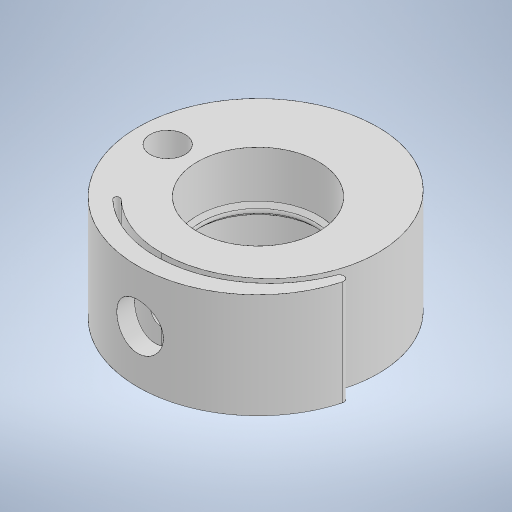
# Autodesk Inventor part: Spool
Saved by Autodesk Inventor 2023.4 (Build 274418000, 418)
## iProperties
Created: 2024-05-13
Part Number: Spool
Material: Generic
Document SubType Name: Modeling
Designer: Nathan Cai
Density: 1 g/cm^3
Appearance: Default
Author: Nathan Cai
Autodesk Inventor part; units mm, degrees
ref_plane "YZ Plane" through (0, 0, 0) normal (1, 0, 0) x (0, 1, 0)
ref_plane "XZ Plane" through (0, 0, 0) normal (0, 1, 0) x (-1, 0, 0)
sketch "Sketch1" plane through (0, 0, 0) normal (1, 0, 0) x (0, 1, 0)
  line L0 (0, 0) -> (9, 0)
  line L1 (9, 0) -> (9, -10.3188)
  line L2 (9, -10.3188) -> (0, -10.3188)
  line L3 (0, -10.3188) -> (0, 0)
  line L4 (9, 0) -> (0, 0)
  line L5 (0, 0) -> (0, -5.2)
  line L6 (0, -5.2) -> (9, -5.2)
  line L7 (9, -5.2) -> (9, 0)
  line L8 (5, -5.2) -> (4, -5.2)
  line L9 (4, -5.2) -> (4, -4.7)
  line L10 (4, -4.7) -> (5, -4.7)
  line L11 (5, -4.7) -> (5, -5.2)
  dimension "d0" = 9
  dimension "d1" = 5.2
  dimension "d2" = 10.3187
  dimension "d3" = 0.5
  dimension "d4" = 4
  dimension "d5" = 4
  constraints: 24 end point, 6 parallel, 3 horizontal, 3 perpendicular, 2 point on line
  measures "d0" distance of L1.end L2.end
  measures "d1" distance of L5.end L4.end
  measures "d2" distance between parallel lines of L0 L2
  measures "d3" distance of L8.end L9.end
  measures "d4" distance between parallel lines of L3 L9
  measures "d5" distance between parallel lines of L1 L11
revolve "Revolution1" add sketch "Sketch1" angle 360 about axis through (0, 0, 0) along (0, 1, 0) contours L6 L1 L2 L3 | L9 L10 L11 L6
chamfer "Chamfer1" distance 0.5 angle 45 2 edges at (0, 4, 4.7) (0, 5, 4.7)
fillet "Fillet1" radius 0.25 2 edges at (0, 4.4999, 4.7) (0, 4.5001, 4.7)
sketch "Sketch2" plane through (0, 9, 0) normal (0, 1, 0) x (1, 0, 0)
  circle A0 centre (0, 0) radius 5.2 projected
  line L0 (-5.2, 0) -> (-10.3188, 0) construction
  circle A1 centre (-7.7594, 0) radius 1.5
  circle A2 centre (0, 0) radius 10.3188 projected
  line L1 (0, 0) -> (0, -10.3188) construction
  arc A3 (0, -8.3188) -> (0, 10.3188) centre (0, 1) ccw
  arc A4 (-5.8822, -5.8822) -> (0, -8.3188) centre (0, 0) ccw
  line L2 (-5.8822, -5.8822) -> (-7.2965, -7.2965)
  arc A5 (0, -8.8268) -> (0, 10.8268) centre (0, 1) ccw
  arc A6 (-6.2415, -6.2415) -> (0, -8.8268) centre (0, 0) ccw
  point P0 (8.7585, 5.4558)
  dimension "d11" = 3
  dimension "d14" = 2
  dimension "d15" = 45
  dimension "d22" = 0.508
  constraints: 12 point on circle, 6 end point, 5 centre point, 4 point on line, 2 tangent, 1 concentric, 1 horizontal, 1 horizontal alignment, 1 line through centre, 1 midpoint, 1 vertical, 1 other
  measures "d11" diameter of A1
  measures "d14" distance of L1.end A3.start
  measures "d15" angle of L1 L2
  measures "d22" radial gap between concentric circles of A3 A5
extrude "Extrusion1" cut sketch "Sketch2" against normal through all contours A1 | A2 A5 A6 L2 A4 A3
sketch "Sketch3" plane through (0, 0, 0) normal (0, 0, 1) x (1, 0, 0)
  line L0 (5.2, 9) -> (-5.2, 9) projected
  line L1 (0, 9) -> (0, 0) construction
  circle A0 centre (0, 4.5) radius 1
  dimension "d16" = 2
  constraints: 2 end point, 2 midpoint, 1 centre point, 1 vertical
  measures "d16" diameter of A0
extrude "Extrusion2" cut sketch "Sketch3" along normal through all
fillet "Fillet2" radius 0.4 1 edges at (8.7585, 4.5, -5.4558)
fillet "Fillet3" radius 0.254 2 edges at (-6.2415, 4.5, 6.2415) (-5.8822, 4.5, 5.8822)
ref_plane "Work Plane1" through (0, 0, 11.1125) normal (0, 0, 1) x (1, 0, 0)
sketch "Sketch4" plane through (0, 0, 11.1125) normal (0, 0, 1) x (1, 0, 0)
  line L0 (0, 9) -> (0, 0) construction
  line L1 (0, 0) -> (0, 9)
  circle A0 centre (0, 4.5) radius 2
  dimension "d26" = 4
  constraints: 2 end point, 1 centre point, 1 collinear, 1 midpoint
  measures "d26" diameter of A0
extrude "Extrusion3" cut sketch "Sketch4" against normal up to surface round surface about axis through (0, 9, 0) along (0, -1, 0) radius 8.8268 far side no
equation "\"d5\" = d4"
body "Solid1"
